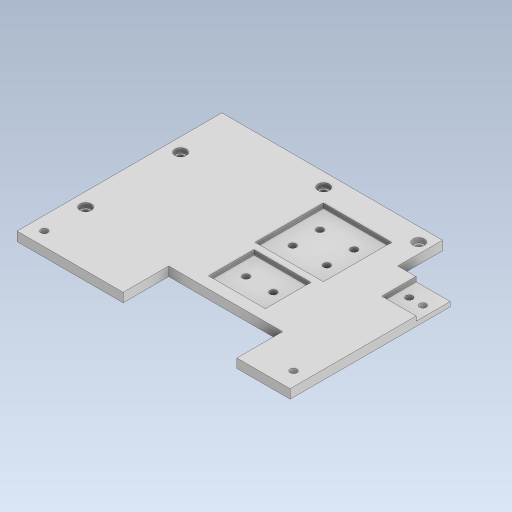
# Autodesk Inventor part: Casis Kiri Bawah
Saved by Autodesk Inventor 2023.5 (Build 275446000, 446)
## iProperties
Created: 2025-09-16
Part Number: Casis Kiri Bawah
Material: Generic
Document SubType Name: Modeling
Designer: Guntur
Density: 1 g/cm^3
Appearance: Default
Author: Guntur
Autodesk Inventor part; units mm, degrees
ref_plane "YZ Plane" through (0, 0, 0) normal (1, 0, 0) x (0, 1, 0)
ref_plane "XZ Plane" through (0, 0, 0) normal (0, 1, 0) x (-1, 0, 0)
ref_plane "XY Plane" through (0, 0, 0) normal (0, 0, 1) x (1, 0, 0)
sketch "Sketch1" plane through (0, 0, 0) normal (0, 1, 0) x (-1, 0, 0)
  line L0 (-61.75, -42) -> (-61.75, 48)
  line L1 (-0.875, 23) -> (-0.875, 3)
  circle A0 centre (-7.375, 13) radius 1.5
  line L2 (11.625, 48) -> (11.625, 28)
  circle A1 centre (-19.375, 13) radius 1.5
  line L3 (-0.875, 3) -> (-25.875, 3)
  line L4 (-25.875, 23) -> (-0.875, 23)
  line L5 (-25.875, 3) -> (-25.875, 23)
  line L6 (-61.75, 48) -> (58.25, 48)
  line L7 (11.625, 28) -> (-38.375, 28)
  line L8 (-38.375, 48) -> (11.625, 48)
  circle A2 centre (-55.75, 40.5) radius 1.5
  line L9 (-38.375, 28) -> (-38.375, 48)
  line L10 (-28.375, 0) -> (-13.375, 0)
  line L11 (-13.375, 0) -> (-13.375, -30)
  line L12 (-13.375, -30) -> (-28.375, -30)
  line L13 (-28.375, -30) -> (-28.375, 0)
  line L14 (1.625, 0) -> (-13.375, 0)
  circle A3 centre (-5.875, -9) radius 1.5
  circle A4 centre (-5.875, -21) radius 1.5
  circle A5 centre (-20.875, -9) radius 1.5
  line L15 (1.625, -30) -> (1.625, 0)
  line L16 (-13.375, 0) -> (-13.375, -30)
  line L17 (-13.375, -30) -> (1.625, -30)
  circle A6 centre (-20.875, -21) radius 1.5
  line L18 (-46.75, -7.35) -> (-61.75, -7.35)
  circle A7 centre (-51.25, -14.85) radius 1.5
  circle A8 centre (-51.25, -14.85) radius 2.5
  circle A9 centre (-57.25, -14.85) radius 1.5
  circle A10 centre (-57.25, -14.85) radius 2.5
  line L19 (-46.75, -22.35) -> (-46.75, -7.35)
  line L20 (-61.75, -7.35) -> (-61.75, -22.35)
  line L21 (-61.75, -22.35) -> (-46.75, -22.35)
  line L22 (-61.75, -25) -> (-61.75, -42)
  line L23 (-61.75, -42) -> (-46.75, -42)
  line L24 (58.25, 48) -> (58.25, -42)
  line L25 (58.25, -42) -> (9.2875, -42)
  circle A11 centre (52.25, 42) radius 1.5
  circle A12 centre (52.25, -17.875) radius 1.5
  circle A13 centre (52.25, -17.875) radius 2.5
  line L26 (43.975, 3) -> (63.025, 3) construction
  circle A14 centre (52.25, 23.875) radius 2.5
  circle A15 centre (52.25, 23.875) radius 1.5
  line L27 (-0.7125, -42) -> (-61.75, -42)
  circle A16 centre (-34.25, -36) radius 2.5
  circle A17 centre (-34.25, -36) radius 1.5
  line L28 (-0.7125, -42) -> (9.2875, -42)
  circle A18 centre (7.5, -36) radius 1.5
  circle A19 centre (7.5, -36) radius 2.5
  line L29 (-13.375, 3) -> (-13.375, -33.5) construction
  line L30 (-46.75, -22.35) -> (-38.75, -22.35)
  line L31 (-38.75, -22.35) -> (-38.75, -42)
  point P0 (6.919, -15.2883)
  point P1 (4.2875, 3)
  point P2 (-0.875, 13)
  point P3 (-34.25, -30)
  point P4 (7.5, -30)
  point P5 (-41.75, -42)
  dimension "d32" = 7.5
  dimension "d33" = 12
  dimension "d34" = 12
  dimension "d35" = 7.5
  dimension "d36" = 0
  dimension "d37" = 0
  dimension "d39" = 8
  constraints: 64 end point, 20 centre point, 6 coincident, 3 point on line, 2 vertical, 1 horizontal, 1 midpoint, 1 perpendicular
  measures "d32" distance from line of L15 A4.centre
  measures "d33" distance of A3.centre A4.centre
  measures "d34" distance of A5.centre A6.centre
  measures "d35" distance from line of L13 A6.centre
  measures "d36" distance between parallel lines of L29 L16
  measures "d37" distance between parallel lines of L29 L11
  measures "d39" distance of L19.start L30.end
extrude "Extrusion1" add sketch "Sketch1" along normal blind 4 contours L31 L30 L19 L18 L0 L6 L9 L7 L2 L24 L25 L28 L27
extrude "Extrusion2" add sketch "Sketch1" along normal blind 2 contours L0 L18 L19 L21 | L1 L3 L5 L4 | L10 L11 L12 L13 | L14 L15 L17 L11 | A8 | A10 | A13 | A14 | A16 | A19
body "Solid1"
